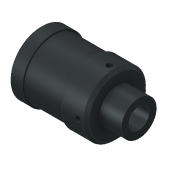
# Autodesk Inventor part: 05.01.006
Saved by Autodesk Inventor 2019.3 (Build 233278000, 278)
## iProperties
Created: 2018-07-09
Part Number: 05.01.006
Material: Чугун, серый
Document SubType Name: Modeling
Designer: MSI-PC
Mass: 927.802 g
Surface Area: 365.172 cm^2
Volume: 129.762 cm^3
Density: 7.15 g/cm^3
Appearance: Чугун серый
Description: Стакан
Author: MSI-PC
Title: Стакан
Autodesk Inventor part; units mm, degrees
ref_plane "YZ Plane" through (0, 0, 0) normal (1, 0, 0) x (0, 1, 0)
ref_plane "XY Plane" through (0, 0, 0) normal (0, 0, 1) x (1, 0, 0)
sketch "Эскиз1" plane through (0, 0, 0) normal (0, 0, 1) x (1, 0, 0)
  line L0 (0, 0) -> (100, 0)
  line L1 (0, 20) -> (0, 32)
  line L2 (0, 32) -> (13, 32)
  line L3 (13, 32) -> (13, 30)
  line L4 (13, 30) -> (53, 30)
  line L5 (53, 30) -> (53, 32)
  line L6 (53, 32) -> (78, 32)
  line L7 (78, 32) -> (78, 18)
  line L8 (78, 18) -> (100, 18)
  line L9 (100, 18) -> (100, 10.5)
  line L10 (100, 10.5) -> (70, 10.5)
  line L11 (70, 10.5) -> (70, 19)
  line L12 (70, 19) -> (64, 19)
  line L13 (64, 19) -> (64, 24.6)
  line L14 (0, 20) -> (56, 20)
  line L15 (56, 20) -> (60.8828, 24.8828)
  line L16 (61.1657, 25) -> (63.6, 25)
  arc A0 (61.1657, 25) -> (60.8828, 24.8828) centre (61.1657, 24.6) ccw
  arc A1 (64, 24.6) -> (63.6, 25) centre (63.6, 24.6) ccw
  point P0 (64, 25)
  point P1 (61, 25)
  dimension "d2" = 100
  dimension "d3" = 40
  dimension "d4" = 25
  dimension "d5" = 22
  dimension "d6" = 21
  dimension "d7" = 36
  dimension "d11" = 38
  dimension "d12" = 6
  dimension "d13" = 64
  dimension "d14" = 64
  dimension "d15" = 60
  dimension "d16" = 45
  dimension "d18" = 3
  dimension "d19" = 0.4
  dimension "d20" = 50
  dimension "d21" = 40
  constraints: 34 end point, 10 perpendicular, 6 point on line, 4 point on circle, 4 tangent, 3 horizontal, 2 centre point, 1 equal radius, 1 parallel, 1 vertical, 1 vertical alignment
  measures "d2" distance between parallel lines of L9 L1
  measures "d3" distance of L3.end L4.end
  measures "d4" distance between parallel lines of L7 L5
  measures "d5" distance of L7.end L8.end
  measures "d6" diameter of L10 L0
  measures "d7" diameter of L8 L0
  measures "d11" diameter of L12 L0
  measures "d12" distance of L11.end L12.end
  measures "d13" distance between parallel lines of L1 L13
  measures "d14" diameter of L2 L0
  measures "d15" diameter of L4 L0
  measures "d16" angle of L16 L15
  measures "d18" distance from line of L13 point (61, 25)
  measures "d19" radius of A0
  measures "d20" diameter of L16 L0
  measures "d21" diameter of L14 L0
revolve "Вращение1" add sketch "Эскиз1" angle 360 about axis through (0, 0, 0) along (1, 0, 0)
sketch "Эскиз2" plane through (0, 0, 0) normal (-1, 0, 0) x (0, 0, 1)
  circle A0 centre (0, 0) radius 32 projected
  constraints: 1 coincident
hole "Отверстие1" at (0, 0, 0) direction (1, 0, 0) diameter 46.376 depth 61 thread size "M48x1.5" class "6H" standard "ISO Metric profile"
ref_plane "РабПлоскость1" through (65.5, 32, 0) normal (0, 1, 0) x (-1, 0, 0)
sketch "Эскиз3" plane through (65.5, 32, 0) normal (0, 1, 0) x (-1, 0, 0)
  line L0 (-12.5, 32) -> (-12.5, -32) projected
  point P0 (65.5, 0)
  point P1 (-4.5, 0)
  dimension "d29" = 8
  constraints: 1 horizontal alignment
  measures "d29" distance from line of L0 point (-4.5, 0)
hole "Отверстие2" at (70, 32, 0) direction (0, -1, 0) diameter 6 depth 5 tip angle 118
pattern_circular "Круговой массив1" count 4 over 360 about axis through (65.5, 0, 0) along (1, 0, 0) of "Отверстие2"
chamfer "Фаска1" distance 3 angle 45 1 edges at (78, -32, 0)
chamfer "Фаска2" distance 1 angle 45 1 edges at (0, -32, 0)
